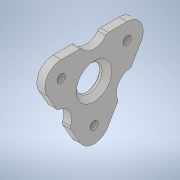
# Autodesk Inventor part: Torque_Triangle
Saved by Autodesk Inventor 2021 (Build 250183000, 183)
## iProperties
Created: 2020-10-13
Part Number: Torque_Triangle
Material: Generic
Document SubType Name: Modeling
Designer: PhotonUser
Density: 1 g/cm^3
Appearance: Default
Author: PhotonUser
Autodesk Inventor part; units mm, degrees
ref_plane "YZ Plane" through (0, 0, 0) normal (1, 0, 0) x (0, 1, 0)
ref_plane "XZ Plane" through (0, 0, 0) normal (0, 1, 0) x (-1, 0, 0)
ref_plane "XY Plane" through (0, 0, 0) normal (0, 0, 1) x (1, 0, 0)
sketch "Sketch1" plane through (0, 0, 0) normal (1, 0, 0) x (0, 1, 0)
  circle A0 centre (0, 0) radius 15.875
  circle A1 centre (18.7452, -32.4676) radius 4.0043
  circle A2 centre (18.7452, -32.4676) radius 15.875
  circle A3 centre (-37.4904, 0) radius 4.0043
  circle A4 centre (-37.4904, 0) radius 15.875
  circle A5 centre (18.7452, 32.4676) radius 15.875
  circle A6 centre (18.7452, 32.4676) radius 4.0043
  circle A7 centre (18.7452, -32.4676) radius 4.0043
  circle A8 centre (18.7452, -32.4676) radius 15.875
  circle A9 centre (0, 0) radius 15.875
  circle A10 centre (-37.4904, 0) radius 4.0043
  circle A11 centre (-37.4904, 0) radius 15.875
  circle A12 centre (18.7452, 32.4676) radius 4.0043
  circle A13 centre (18.7452, 32.4676) radius 15.875
  line L0 (34.6202, 32.4676) -> (34.6202, -32.4676)
  line L1 (10.8077, -46.2158) -> (-45.4279, -13.7482)
  line L2 (10.8077, 46.2158) -> (-45.4279, 13.7482)
  circle A14 centre (18.7452, 32.4676) radius 15.875
  circle A15 centre (-37.4904, 0) radius 15.875
  circle A16 centre (18.7452, -32.4676) radius 15.875
  circle A17 centre (41.995, 0) radius 14.4142
  circle A18 centre (-20.9975, 36.3687) radius 14.4142
  circle A19 centre (-20.9975, -36.3687) radius 14.4142
  point P0 (-28.0356, -23.7896)
  point P1 (-6.5846, -36.1743)
  point P2 (10.8077, -46.2158)
  point P3 (34.6202, -12.3847)
  point P4 (34.6202, 12.3847)
  point P5 (-6.5846, 36.1743)
  point P6 (-28.0356, 23.7896)
  point P7 (-45.4279, 13.7482)
  point P8 (-45.4279, -13.7482)
  dimension "d28" = 360
  dimension "d34" = 31.75
  dimension "d35" = 28.8284
  dimension "d36" = 8.0086
  dimension "d37" = 31.75
  dimension "d38" = 31.75
  dimension "d39" = 60
  dimension "d40" = 60
  dimension "d41" = 7.3748
  dimension "d42" = 55.6177
  dimension "d43" = 55.6177
  dimension "d44" = 0
  dimension "d45" = 41.2048
  dimension "d46" = 0
  dimension "d47" = 62.6558
  dimension "d48" = 80.0481
  dimension "d49" = 0
  dimension "d50" = 80.0481
  dimension "d51" = 15.875
  dimension "d52" = 15.875
  dimension "d53" = 23.8125
  dimension "d54" = 80.0481
  dimension "d55" = 34.6202
  dimension "d56" = 34.6202
  dimension "d57" = 41.2048
  dimension "d58" = 0
  dimension "d59" = 41.2048
  dimension "d60" = 62.6558
  dimension "d61" = 62.6558
  dimension "d62" = 0
  dimension "d63" = 62.6558
  dimension "d64" = 41.2048
  dimension "d65" = 72.1106
  dimension "d66" = 80.0481
  dimension "d67" = 0
  dimension "d68" = 80.0481
  dimension "d69" = 23.8125
  constraints: 20 centre point, 12 equal radius, 9 tangent, 8 coincident, 6 end point, 6 point on circle, 3 concentric, 1 vertical, 7 other
  measures "d34" diameter of A0
  measures "d35" diameter of A17
  measures "d36" diameter of A6
  measures "d37" diameter of A8
  measures "d38" diameter of A15
  measures "d39" angle of L2 L0
  measures "d40" angle of L1 L0
  measures "d41" distance from line of A17.centre L0
  measures "d42" distance from line of A17.centre L2
  measures "d43" distance from line of A17.centre L1
  measures "d44" distance from line of point (34.62, 12.385) L0
  measures "d45" distance from line of point (34.62, 12.385) L2
  measures "d46" distance from line of point (34.62, -12.385) L0
  measures "d47" distance from line of point (34.62, -12.385) L2
  measures "d48" distance from line of L0.end L2
  measures "d49" distance from line of point (34.62, -32.468) L0
  measures "d50" distance from line of point (34.62, -32.468) L2
  measures "d51" distance from line of A5.centre L0
  measures "d52" distance from line of A5.centre L2
  measures "d53" distance from line of point (10.808, -46.216) L0
  measures "d54" distance from line of point (10.808, -46.216) L2
  measures "d55" distance from line of A9.centre L0
  measures "d56" distance from line of A9.centre L2
  measures "d57" distance from line of point (-6.585, 36.174) L0
  measures "d58" distance from line of point (-6.585, 36.174) L2
  measures "d59" distance from line of point (-6.585, -36.174) L0
  measures "d60" distance from line of point (-6.585, -36.174) L2
  measures "d61" distance from line of point (-28.036, 23.79) L0
  measures "d62" distance from line of point (-28.036, 23.79) L2
  measures "d63" distance from line of point (-28.036, -23.79) L0
  measures "d64" distance from line of point (-28.036, -23.79) L2
  measures "d65" distance from line of A15.centre L0
  measures "d66" distance from line of point (-45.428, 13.748) L0
  measures "d67" distance from line of point (-45.428, 13.748) L2
  measures "d68" distance from line of point (-45.428, -13.748) L0
  measures "d69" distance from line of point (-45.428, -13.748) L2
extrude "Extrusion1" add sketch "Sketch1" along normal blind 7.9375 contours A2 | A2 L1 A19 A4 L2 A18 A5 L0 A17 | A5 | A4
fillet "Fillet2" radius 3.175 6 edges at (3.9688, 34.6202, 12.3847) (3.9688, 34.6202, -12.3847) (3.9688, -6.5846, 36.1743) (3.9688, -28.0356, 23.7896) (3.9688, -6.5846, -36.1743) (3.9688, -28.0356, -23.7896)
sketch "Sketch5" plane through (7.9375, 0, 0) normal (1, 0, 0) x (0, 0, -1)
  circle A0 centre (0, 0) radius 15.875
  circle A1 centre (0, 0) radius 12.7
  dimension "d70" = 25.4
  constraints: 2 centre point, 2 coincident
  measures "d70" diameter of A1
extrude "Extrusion3" add sketch "Sketch5" against normal up to surface (7.9375 mm away)
chamfer "Chamfer5" distance 4.7625 angle 45 1 edges at (7.9375, 0, 12.7)
chamfer "Chamfer7" distance 0.762 angle 45 1 edges at (0, 0, 12.7)
body "Solid1"
